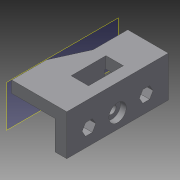
# Autodesk Inventor part: world_cam_mount
Saved by Autodesk Inventor 2015 (Build 190159000, 159)
## iProperties
Created: 2015-06-20
Part Number: world_cam_mount
Material: Generic
Document SubType Name: Modeling
Designer: Master
Density: 1 g/cm^3
Appearance: Default
Author: Master
Autodesk Inventor part; units mm, degrees
ref_plane "YZ Plane" through (0, 0, 0) normal (1, 0, 0) x (0, 1, 0)
ref_plane "XZ Plane" through (0, 0, 0) normal (0, 1, 0) x (-1, 0, 0)
ref_plane "XY Plane" through (0, 0, 0) normal (0, 0, 1) x (1, 0, 0)
sketch "Sketch1" plane through (0, 0, 0) normal (0, 1, 0) x (-1, 0, 0)
  line L0 (4.6826, 5.0563) -> (-4.3174, 5.0563)
  line L1 (-4.3174, 5.0563) -> (-4.3174, -5.9437)
  line L2 (-4.3174, -5.9437) -> (-0.3174, -5.9437)
  line L3 (4.6826, 5.0563) -> (-0.3174, -5.9437)
  point P0 (0, 0)
  dimension "d0" = 11
  dimension "d1" = 9
  dimension "d2" = 4
  constraints: 8 end point
  measures "d0" distance between parallel lines of L2 L0
  measures "d1" distance of L0.start L0.end
  measures "d2" distance of L1.end L2.end
extrude "Extrusion1" add sketch "Sketch1" along normal blind 10
sketch "Sketch2" plane through (4.3174, 0, 5.0563) normal (1, 0, 0) x (0, 0, -1)
  line L0 (5.5037, 7.3678) -> (7.55, 3.815)
  line L1 (7.55, 3.815) -> (5.4963, 2.6322)
  line L2 (5.4963, 2.6322) -> (3.45, 6.185)
  line L3 (3.45, 6.185) -> (5.5037, 7.3678)
  line L4 (3.45, 6.185) -> (7.55, 6.185)
  line L5 (7.55, 6.185) -> (7.55, 3.815)
  line L6 (7.55, 3.815) -> (3.45, 3.815)
  line L7 (3.45, 3.815) -> (3.45, 6.185)
  line L8 (5.5037, 7.3678) -> (7.55, 6.185)
  line L9 (3.45, 3.815) -> (5.4963, 2.6322)
  line L10 (0, 0) -> (11, 0) projected
  line L11 (11, 0) -> (11, 10) projected
  line L12 (0, 10) -> (11, 10) projected
  line L13 (0, 0) -> (0, 10) projected
  line L14 (3.45, 6.185) -> (7.55, 3.815)
  line L15 (3.45, 3.815) -> (7.55, 6.185)
  line L16 (5.5037, 7.3678) -> (5.4963, 2.6322)
  point P0 (5.0563, 0)
  point P1 (11, 0)
  point P2 (5.5, 5)
  dimension "d6" = 4.1
  dimension "d7" = 2.37
  dimension "d8" = 4.1
  dimension "d9" = 2.37
  dimension "d11" = 5
  dimension "d12" = 5.5
  constraints: 26 end point, 1 midpoint, 1 perpendicular
  measures "d6" distance between parallel lines of L1 L3
  measures "d7" distance between parallel lines of L0 L2
  measures "d8" distance between parallel lines of L5 L7
  measures "d9" distance between parallel lines of L6 L4
  measures "d11" distance from line of L12 point (5.5, 5)
  measures "d12" distance from line of L11 point (5.5, 5)
extrude "Extrusion2" cut sketch "Sketch2" against normal through all contours L8 L4 L0 | L16 L4 L3 | L0 L4 L16 | L4 L15 L0 | L0 L15 L16 L4 | L14 L15 L2 | L2 L15 L7 | L4 L16 L14 | L5 L0 L15 | L0 L14 L15 | L15 L16 L6 L2 | L2 L6 L15 | L6 L2 L9 | L14 L6 L16 | L1 L16 L6 | L6 L16 L2
sketch "Sketch3" plane through (0, 10, 0) normal (0, 1, 0) x (1, 0, 0)
  line L0 (-4.6826, -5.0563) -> (4.3174, -5.0563) projected
  line L1 (4.3174, -5.0563) -> (4.3174, 5.9437) projected
  line L2 (4.3174, 5.9437) -> (0.3174, 5.9437) projected
  line L3 (0.3174, 5.9437) -> (-4.6826, -5.0563) projected
  line L4 (0.3399, 17.9475) -> (4.3174, 17.9475)
  line L5 (4.3174, 17.9475) -> (4.3174, -17.0525)
  line L6 (4.3174, -17.0525) -> (0.3399, -17.0525)
  line L7 (0.3399, -17.0525) -> (0.3399, 17.9475)
  line L8 (4.3174, -1.6063) -> (-3.1144, -1.6063) projected
  line L9 (4.3174, 2.4937) -> (-1.2508, 2.4937) projected
  line L10 (4.3174, 0.4475) -> (-2.1809, 0.4475) projected
  line L11 (4.3174, 17.9475) -> (14.3174, 17.9475)
  line L12 (14.3174, 17.9475) -> (14.3174, -17.0525)
  line L13 (14.3174, -17.0525) -> (4.3174, -17.0525)
  line L14 (4.3174, -17.0525) -> (4.3174, 17.9475)
  line L15 (4.3174, 6.4475) -> (10.3174, 6.4475)
  line L16 (10.3174, 6.4475) -> (10.3174, -5.5525)
  line L17 (10.3174, -5.5525) -> (4.3174, -5.5525)
  line L18 (4.3174, -5.5525) -> (4.3174, 6.4475)
  point P0 (0, 0)
  dimension "d15" = 35
  dimension "d16" = 17.5
  dimension "d17" = 10
  dimension "d18" = 6
  dimension "d19" = 6
  dimension "d20" = 12
  constraints: 24 end point, 2 collinear, 1 point on line, 1 vertical
  measures "d15" distance between parallel lines of L4 L6
  measures "d16" distance between parallel lines of L10 L6
  measures "d17" distance between parallel lines of L14 L12
  measures "d18" distance between parallel lines of L5 L16
  measures "d19" distance between parallel lines of L10 L17
  measures "d20" distance between parallel lines of L15 L17
extrude "Extrusion3" add sketch "Sketch3" along normal blind 1 contours L3 L8 L7 L0 | L7 L8 L1 L0 | L0 L5 L6 L7 | L3 L10 L7 L8 | L7 L10 L1 L8 | L3 L9 L7 L10 | L17 L16 L15 L5 L11 L12 L13 | L7 L9 L1 L10 | L3 L2 L7 L9 | L7 L2 L1 L9 | L7 L4 L5 L2
sketch "Sketch4" plane through (0, 10, 0) normal (0, -1, 0) x (1, 0, 0)
  line L0 (4.3174, -5.9437) -> (0.3399, -5.9437) projected
  line L1 (0.3399, -17.9475) -> (0.3399, -5.9437) projected
  line L2 (14.3174, -17.9475) -> (0.3399, -17.9475) projected
  line L3 (14.3174, 17.0525) -> (14.3174, -17.9475) projected
  line L4 (0.3399, 17.0525) -> (14.3174, 17.0525) projected
  line L5 (0.3399, 5.0563) -> (0.3399, 17.0525) projected
  line L6 (0.3399, 5.0563) -> (4.3174, 5.0563) projected
  line L7 (4.3174, 5.0563) -> (4.3174, 5.5525) projected
  line L8 (4.3174, 5.5525) -> (10.3174, 5.5525) projected
  line L9 (10.3174, 5.5525) -> (10.3174, -6.4475) projected
  line L10 (10.3174, -6.4475) -> (4.3174, -6.4475) projected
  line L11 (4.3174, -6.4475) -> (4.3174, -5.9437) projected
  line L12 (0.3399, 17.0525) -> (14.3174, 17.0525) projected
  line L13 (14.3174, -17.9475) -> (10.3174, -17.9475)
  line L14 (10.3174, -17.9475) -> (10.3174, 17.0525)
  line L15 (10.3174, 17.0525) -> (14.3174, 17.0525)
  line L16 (14.3174, 17.0525) -> (14.3174, -17.9475)
  point P0 (0, 0)
  dimension "d23" = 4
  constraints: 8 end point, 1 point on line
  measures "d23" distance between parallel lines of L3 L14
extrude "Extrusion4" add sketch "Sketch4" along normal blind 10 contours L9 L14 L4 L3 L2
sketch "Sketch5" plane through (14.3174, 11, 17.0525) normal (1, 0, 0) x (0, 0, -1)
  line L0 (5.2643, -5.4963) -> (8.8172, -3.45)
  line L1 (8.8172, -3.45) -> (10, -5.5037)
  line L2 (10, -5.5037) -> (6.4472, -7.55)
  line L3 (6.4472, -7.55) -> (5.2643, -5.4963)
  line L4 (6.4472, -7.55) -> (6.4472, -3.45)
  line L5 (6.4472, -3.45) -> (8.8172, -3.45)
  line L6 (8.8172, -3.45) -> (8.8172, -7.55)
  line L7 (8.8172, -7.55) -> (6.4472, -7.55)
  line L8 (5.2643, -5.4963) -> (6.4472, -3.45)
  line L9 (8.8172, -7.55) -> (10, -5.5037)
  line L10 (19.2733, 12.7) -> (12, 12.7)
  line L11 (25, -5.5037) -> (28.5528, -3.4574)
  line L12 (28.5528, -3.4574) -> (29.7357, -5.5112)
  line L13 (29.7357, -5.5112) -> (26.1828, -7.5574)
  line L14 (26.1828, -7.5574) -> (25, -5.5037)
  line L15 (26.1828, -7.5574) -> (26.1828, -3.4574)
  line L16 (26.1828, -3.4574) -> (28.5528, -3.4574)
  line L17 (28.5528, -3.4574) -> (28.5528, -7.5574)
  line L18 (28.5528, -7.5574) -> (26.1828, -7.5574)
  line L19 (25, -5.5037) -> (26.1828, -3.4574)
  line L20 (28.5528, -7.5574) -> (29.7357, -5.5112)
  line L21 (0, 0) -> (35, 0) projected
  line L22 (0, 0) -> (0, -11) projected
  line L23 (35, -11) -> (35, 0) projected
  line L24 (6.4472, -7.55) -> (8.8172, -3.45)
  line L25 (6.4472, -3.45) -> (8.8172, -7.55)
  line L26 (10, -5.5037) -> (5.2643, -5.4963)
  line L27 (26.1828, -3.4574) -> (28.5528, -7.5574)
  line L28 (26.1828, -7.5574) -> (28.5528, -3.4574)
  line L29 (25, -5.5037) -> (29.7357, -5.5112)
  line L30 (35, -11) -> (35, 0) projected
  line L31 (0, 0) -> (35, 0) projected
  line L32 (0, 0) -> (0, -11) projected
  line L33 (35, -11) -> (0, -11) projected
  line L34 (19.5463, -7.185) -> (17.4926, -8.3678) projected
  line L35 (17.4926, -8.3678) -> (15.4463, -7.185) projected
  line L36 (15.4463, -7.185) -> (15.4463, -4.815) projected
  line L37 (15.4463, -4.815) -> (17.5, -3.6322) projected
  line L38 (17.5, -3.6322) -> (19.5463, -4.815) projected
  line L39 (19.5463, -4.815) -> (19.5463, -7.185) projected
  line L40 (15.4463, -7.185) -> (19.5463, -4.815)
  line L41 (15.4463, -4.815) -> (19.5463, -7.185)
  line L42 (19.5463, -7.185) -> (17.4926, -8.3678)
  line L43 (17.5, -3.6322) -> (17.4926, -8.3678)
  circle A0 centre (17.4963, -6) radius 1.5
  point P0 (17.0525, -11)
  point P1 (11, 0)
  point P2 (7.6322, -5.5)
  point P3 (27.3678, -5.5074)
  dimension "d26" = 4.1
  dimension "d27" = 2.37
  dimension "d28" = 4.1
  dimension "d29" = 2.37
  dimension "d31" = 4.1
  dimension "d32" = 2.37
  dimension "d33" = 4.1
  dimension "d34" = 2.37
  dimension "d36" = 10
  dimension "d37" = 10
  dimension "d38" = 5.5
  dimension "d39" = 3
  constraints: 62 end point, 3 midpoint, 2 parallel, 2 perpendicular, 1 centre point, 1 coincident, 1 horizontal alignment
  measures "d26" distance between parallel lines of L1 L3
  measures "d27" distance between parallel lines of L0 L2
  measures "d28" distance between parallel lines of L5 L7
  measures "d29" distance between parallel lines of L6 L4
  measures "d31" distance between parallel lines of L12 L14
  measures "d32" distance between parallel lines of L11 L13
  measures "d33" distance between parallel lines of L16 L18
  measures "d34" distance between parallel lines of L17 L15
  measures "d36" distance from line of L1.end L22
  measures "d37" distance from line of L11.start L23
  measures "d38" distance from line of point (7.632, -5.5) L21
  measures "d39" diameter of A0
extrude "Extrusion5" cut sketch "Sketch5" against normal up to surface (4 mm away) contours L8 L4 L0 | L26 L4 L3 | L0 L4 L26 | L4 L25 L0 | L0 L25 L26 L4 | L24 L25 L2 | L2 L25 L7 | L4 L26 L24 | L5 L0 L25 | L0 L24 L25 | L25 L26 L6 L2 | L2 L6 L25 | L6 L2 L9 | L24 L6 L26 | L1 L26 L6 | L6 L26 L2 | L19 L15 L11 | L29 L15 L14 | L11 L15 L29 | L15 L27 L11 | L11 L27 L29 L15 | L28 L27 L13 | L13 L27 L18 | L15 L29 L28 | L16 L11 L27 | L11 L28 L27 | L27 L29 L17 L13 | L13 L17 L27 | L17 L13 L20 | L28 L17 L29 | L12 L29 L17 | L17 L29 L13 | A0 L43 L41 | L41 L40 A0 | A0 L40 L43 | L40 L43 A0 | L40 A0 L41 | L41 A0 L43
sketch "Sketch6" plane through (14.3174, 11, 17.0525) normal (1, 0, 0) x (0, 0, -1)
  circle A0 centre (17.4963, -6) radius 1.5 projected
  circle A1 centre (17.4963, -6) radius 3
  point P0 (17.0525, -11)
  dimension "d42" = 6
  constraints: 1 centre point, 1 coincident
  measures "d42" diameter of A1
extrude "Extrusion6" cut sketch "Sketch6" against normal blind 2
sketch "Sketch7" plane through (0, 11, 0) normal (0, 1, 0) x (1, 0, 0)
  line L0 (4.3174, 6.4475) -> (4.3174, -5.5525) projected
  line L1 (4.3174, 6.4475) -> (10.3174, 6.4475) projected
  line L2 (10.3174, 6.4475) -> (10.3174, -5.5525) projected
  line L3 (10.3174, -5.5525) -> (4.3174, -5.5525) projected
  line L4 (0.3399, 5.9437) -> (0.3174, 5.9437) projected
  line L5 (0.3174, 5.9437) -> (-4.6826, -5.0563) projected
  line L6 (-4.6826, -5.0563) -> (0.3399, -5.0563) projected
  line L7 (0.3399, -5.0563) -> (0.3399, -17.0525) projected
  line L8 (0.3399, -17.0525) -> (14.3174, -17.0525) projected
  line L9 (14.3174, -17.0525) -> (14.3174, 17.9475) projected
  line L10 (14.3174, 17.9475) -> (0.3399, 17.9475) projected
  line L11 (0.3399, 17.9475) -> (0.3399, 5.9437) projected
  point P0 (0, 0)
extrude "Extrusion7" add sketch "Sketch7" along normal blind 3
ref_plane "Work Plane1" through (-4.6826, 7, 5.0563) normal (-1, 0, 0) x (0, 0, 1)
sketch "Sketch8" plane through (-4.6826, 7, 5.0563) normal (-1, 0, 0) x (0, 0, 1)
  circle A0 centre (-5.5, -2) radius 3 projected
  circle A1 centre (-5.5, -2) radius 4.211
  point P0 (-5.0563, -7)
  constraints: 1 centre point, 1 coincident
extrude "Extrusion8" cut sketch "Sketch8" against normal blind 3 contours A0 | A1
sketch "Sketch9" plane through (0.3399, 10, 5.0563) normal (-1, 0, 0) x (0, 0, 1)
  line L0 (0, 0) -> (0, 4) projected
  line L1 (0, 0) -> (11.9963, 0) projected
  line L2 (11.9963, 0) -> (11.9963, 4) projected
  line L3 (0, 4) -> (11.9963, 4) projected
  point P0 (-5.0563, -10)
extrude "Extrusion9" add sketch "Sketch9" along normal up to surface (5.0225 mm away)
equation "\"d16\" = 0.5 * d15"
body "Solid1"
